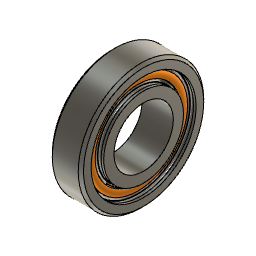
bearing v1 (Autodesk Fusion 360 design; units mm, degrees)
Autodesk Fusion 360 part; units mm, degrees
sketch "Sketch1" plane through (0, 0, 0) normal (0, 0, 1) x (1, 0, 0)
  line L0 (-59.5, 63) -> (59.5, 63)
  line L1 (59.5, -63) -> (-59.5, -63)
  line L2 (-37.5, 22) -> (0, 22)
  line L3 (-37.5, 24) -> (-37.5, 22)
  arc A0 (-37.5, 24) -> (-49.5, 24) centre (-43.5, 24) ccw
  line L4 (-59.5, 24) -> (-49.5, 24)
  line L5 (0, 0) -> (0, 50.1937) construction
  line L6 (-34, 0) -> (-43.8483, 0) construction
  arc A1 (49.5, 24) -> (37.5, 24) centre (43.5, 24) ccw
  line L7 (59.5, 24) -> (49.5, 24)
  line L8 (37.5, 22) -> (0, 22)
  line L9 (37.5, 24) -> (37.5, 22)
  line L10 (-59.5, -24) -> (-49.5, -24)
  arc A2 (-49.5, -24) -> (-37.5, -24) centre (-43.5, -24) ccw
  line L11 (-37.5, -22) -> (0, -22)
  line L12 (-37.5, -24) -> (-37.5, -22)
  line L13 (37.5, -22) -> (0, -22)
  arc A3 (37.5, -24) -> (49.5, -24) centre (43.5, -24) ccw
  line L14 (59.5, -24) -> (49.5, -24)
  line L15 (37.5, -24) -> (37.5, -22)
  arc A4 (-37.8286, 13) -> (-37.8286, -13) centre (0, 0) ccw
  arc A5 (37.8286, -13) -> (37.8286, 13) centre (0, 0) ccw
  line L16 (-37.8286, 13) -> (37.8286, 13)
  line L17 (-37.8286, -13) -> (37.8286, -13)
  line L18 (-59.5, -63) -> (-59.5, -24)
  line L19 (-59.5, 24) -> (-59.5, 63)
  line L20 (59.5, 63) -> (59.5, 24)
  line L21 (59.5, -24) -> (59.5, -63)
  line L22 (0, -63) -> (0, -176) construction
  line L23 (0, -176) -> (3.6696, -176) construction
  line L24 (3.6696, -176) -> (52.7077, -176) construction
  dimension "d2" = 126
  dimension "d3" = 119
  dimension "d4" = 59.5
  dimension "d5" = 63
  dimension "d6" = 39
  dimension "d7" = 41
  dimension "d8" = 12
  dimension "d9" = 16
  dimension "d10" = 80
  dimension "d11" = 50
  dimension "d12" = 50
  dimension "d13" = 113
  constraint horizontal L0
  constraint vertical L20
  constraint horizontal L1
  constraint vertical L18
  constraint coincident L4.start L18
  constraint perpendicular L4 L20
  constraint perpendicular L2 L20
  constraint coincident A0.centre L4
  constraint tangent L3 A0
  constraint perpendicular L2 L5
  constraint perpendicular L5 L6
  constraint coincident L5 L2.end
  constraint symmetric L4.start L5 L7.start
  constraint symmetric L3.start L5 A1.end
  constraint symmetric A0.end L5 A1.start
  constraint symmetric A0 L5 A1
  constraint symmetric L2.start L5 L8.start
  constraint symmetric L5 L2.end L8.end
  constraint symmetric L4.start L6 L10.start
  constraint symmetric L3.start L6 A2.end
  constraint symmetric A0.end L6 L10.end
  constraint symmetric A0 L6 A2
  constraint symmetric L2.start L6 L11.start
  constraint symmetric L6 L2.end L11.end
  constraint symmetric L6 A1.end A3.start
  constraint symmetric L6 A1.start A3.end
  constraint symmetric L6 A1 A3
  constraint symmetric L6 L7.start L14.start
  constraint symmetric L6 L8.start L13.start
  constraint coincident L5.start A4.centre
  constraint concentric A4 A5
  constraint perpendicular L16 L20
  constraint perpendicular L17 L20
  constraint collinear L18 L19
  constraint collinear L20 L21
  constraint midpoint L1 L22.start
  constraint perpendicular L1 L22
  constraint perpendicular L22 L23
  constraint perpendicular L22 L24
  measures "d2" distance of L0.end L1.start
  measures "d3" distance of L0.start L0.end
  measures "d4" distance of L5.start L20
  measures "d5" distance of L5.start L1
  measures "d6" distance of L0 L4
  measures "d7" distance of L0 L2
  measures "d8" diameter of A0
  measures "d9" distance of A0.centre L18
  measures "d10" diameter of A4
  measures "d11" distance of L0 L16
  measures "d12" distance of L1 L17
  measures "d13" distance of L22.start L22.end
revolve "Revolve1" add sketch "Sketch1" angle 360 about axis through (3.6696, -176, 0) along (1, 0, 0) makes body 1 at (-19.8333, 62.7029, -11.9132) makes body 2 at (-12.6095, 12.7651, -9.4209) makes body 3 at (19.8333, -63.1405, -5.6326)
chamfer "Chamfer1" distance 10 angle 45 1 edges at (-59.5, -262.4261, 222.8262) on bodies 1
chamfer "Chamfer2" distance 10 angle 45 1 edges at (59.5, -262.4261, 222.8262) on bodies 1
sphere "SpherePrimitive1" add diameter 68 placed x (1, 0, 0) y (0, 1, 0) z (0, 0, 1) at (0, 0, 0) separate body makes body 4
pattern_circular "C-Pattern1" count 13 over 360 about axis through (3.6696, -176, 0) along (1, 0, 0) of bodies 4 makes body 5 at (32.2345, -9.6812, 79.1202) makes body 6 at (32.2345, -65.501, 147.3497) makes body 7 at (32.2345, -148.5723, 165.8663) makes body 8 at (32.2345, -234.4958, 174.643) makes body 9 at (32.2345, -296.9246, 116.7954) makes body 10 at (32.2345, -352.9578, 51.0675) makes body 11 at (32.2345, -356.4206, -37.0184) makes body 12 at (32.2345, -306.5197, -105.9648) makes body 13 at (32.2345, -248.025, -169.5121) makes body 14 at (32.2345, -160.9988, -183.5672) makes body 15 at (32.2345, -77.4092, -155.5693) makes body 16 at (32.2345, -16.4055, -91.9323)
combine "Combine1" operation cut target body 2 tool bodies 6 7 8 9 10 11 12 13 14 16 15 4 5
chamfer "Chamfer3" distance 1 angle 45 26 edges at (0, -43.535, 134.811) (0, -109.7732, 148.9396) (0, -121.3579, 180.9288) (0, -186.5747, 162.6566) (0, -211.6986, 185.598) (0, -260.9538, 139.111) (0, -293.8612, 147.7489) (0, -315.8709, 83.6967) (0, -349.0233, 76.0523) (0, -338.7453, 9.1085) (0, -364.5478, -13.0669) (0, -324.3367, -67.5664) (0, -336.8782, -99.1927) (0, -275.946, -128.7626) (0, -204.6588, -160.4608) (0, -272.3534, -162.5946) (0, -126.8063, -155.3994) (0, -185.7552, -188.7481) (0, -60.2234, -114.7379) (0, -96.9222, -171.6616) (0, -20.1636, -47.7913) (0, -26.205, -115.2495) (0, -48.1434, 101.1023) (0, 3.9418, 57.8097) (0, -15.804, 30.1037) (0, 10.196, -32.4352) on bodies 2
sphere "SpherePrimitive2" add diameter 68 placed x (1, 0, 0) y (0, 1, 0) z (0, 0, 1) at (0, 0, 0) separate body makes body 17
pattern_circular "C-Pattern2" count 13 over 360 about axis through (3.6696, -176, 0) along (1, 0, 0) of bodies 17 makes body 18 at (32.2345, -9.6812, 79.1202) makes body 19 at (32.2345, -65.501, 147.3497) makes body 20 at (32.2345, -148.5723, 165.8663) makes body 21 at (32.2345, -234.4958, 174.643) makes body 22 at (32.2345, -296.9246, 116.7954) makes body 23 at (32.2345, -352.9578, 51.0675) makes body 24 at (32.2345, -356.4206, -37.0184) makes body 25 at (32.2345, -306.5197, -105.9648) makes body 26 at (32.2345, -248.025, -169.5121) makes body 27 at (32.2345, -160.9988, -183.5672) makes body 28 at (32.2345, -77.4092, -155.5693) makes body 29 at (32.2345, -16.4055, -91.9323)
